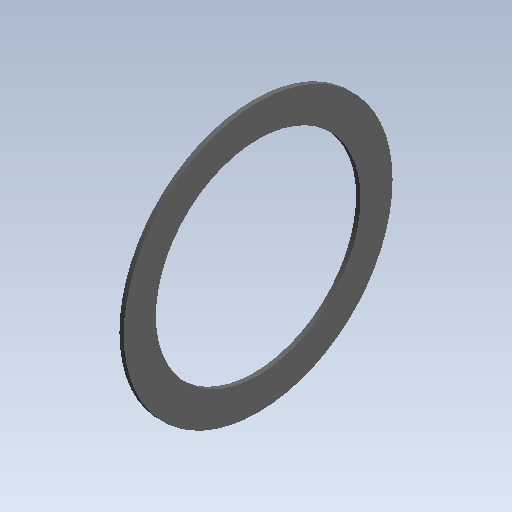
# Autodesk Inventor part: MR106ZZ1 Shield2
Saved by Autodesk Inventor 2021.3 (Build 253353010, 353A)
## iProperties
Part Number: MR106ZZ1 Shield2
Material: 一般
Catalog Web Link: www.cadenas.de
Description: shielde_type_zz_zzs_S2-
Vendor: NSK_RB
Document SubType Name: Modeling
Designer: partserver
Manufacturer: NSK_RB
Mass: 0.00422429 g
Surface Area: 0.641959 cm^2
Volume: 0.00422429 cm^3
Density: 1 g/cm^3
Appearance: PSOLRGB-128-128-128
Category: PARTsolutions
Company: NSK_RB
PSOL_IDENT_0: {$CADENAS_DATA\23d-libs\nsk_rb\roller_bearings\deep_groove_bb\exstra_small_miniatur_bb\metric_design
PSOL_IDENT_1: \shielded_type_zz_zzs_s2.prj},189 {VTYP=3D},{NB=MR106ZZ1 Shield2},{LINA=MR106ZZ1 Shield2},{NN=shield
PSOL_IDENT_2: e_type_zz_zzs_S2},{DATE=25.05.2021 06:41:25},{GEOMDATE=04.01.2008 00:00:00},{VERSION=},{LINEID=600},
PSOL_IDENT_3: {WBVAR=},{WBNUMERIC=}  {NB=MR106ZZ1 Shield2},{LINA=MR106ZZ1 Shield2},{KT=DUMMY},{IDNR=},{STAN=Standa
PSOL_IDENT_4: rd},{ORDER=MR106ZZ1},{SD=6.0},{X=6.0},{DI1=7.04},{DI2=7.04},{SDE1=8.90},{SDE2=9.25},{D=10},{DD=10},{
PSOL_IDENT_5: B=0.0},{B1=3.0},{R=0.00},{R1=0.10},{CR1=495},{COR1=218},{CR2=51},{COR2=22.0},{LG=45000},{LO=53000},{
PSOL_IDENT_6: DA=0.0},{DB=7.0},{DA1=0.0},{DB1=9.3},{RA=0.00},{RB=0.10},{MASS=0.68},{SC=1}
NB: MR106ZZ1 Shield2
NN: shielde_type_zz_zzs_S2
NBSYN: $ORDER. Shield2
LINA: MR106ZZ1 Shield2
CATALOG: NSK Rolling Bearing
STAN: Standard
ORDER: MR106ZZ1
SD: 6
X: 6
DI1: 7.04
DI2: 7.04
SDE1: 8.9
SDE2: 9.25
D: 10
DD: 10
B: 0
B1: 3
R: 0
R1: 0.1
CR1: 495
COR1: 218
CR2: 51
COR2: 22
LG: 45000
LO: 53000
DA: 0
DB: 7
DA1: 0
DB1: 9.3
RA: 0
RB: 0.1
MASS: 0.68
SC: 1
SUPPLIER: NSK_RB
ARTICLENO: MR106ZZ1 Shield2
BOMINFO: MR106ZZ1 Shield2
CREATOR: CADENAS GmbH
Title: MR106ZZ1 Shield2
Author: Cadenas PARTsolutions
Autodesk Inventor part; units mm, degrees
sketch "Sketch_1" plane through (0, 0, 0) normal (0, 0, 1) x (1, 0, 0)
  line L0 (2.9502, 0) -> (2.8008, 0)
  line L1 (2.8008, 3.52) -> (2.9502, 3.52)
  line L2 (2.9502, 3.52) -> (2.9502, 4.625)
  line L3 (2.9502, 4.625) -> (2.8008, 4.625)
  line L4 (2.8008, 4.625) -> (2.8008, 3.52)
  constraints: 10 end point
revolve "Revolution1" add sketch "Sketch_1" angle 360 about axis through (2.9502, 0, 0) along (1, 0, 0)
ref_plane "ip_st_s2_XY" through (2.8008, 0, 0) normal (1, 0, 0) x (0, 0, -1)
ref_plane "ip_st_s2_YZ" through (2.8008, 0, 0) normal (0, 0, -1) x (0, 1, 0)
ref_plane "ip_st_s2_ZX" through (2.8008, 0, 0) normal (0, 1, 0) x (1, 0, 0)
body "Solid1"
